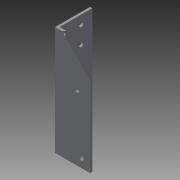
# Autodesk Inventor part: 2x2 angle vertical left
Saved by Autodesk Inventor 2015 (Build 190159000, 159)
## iProperties
Created: 2015-01-16
Part Number: 2x2 angle vertical left
Material: Generic
Document SubType Name: Modeling
Designer: 215152
Density: 1 g/cm^3
Appearance: Default
Author: 215152
Autodesk Inventor part; units mm, degrees
ref_plane "YZ Plane" through (0, 0, 0) normal (1, 0, 0) x (0, 1, 0)
ref_plane "XZ Plane" through (0, 0, 0) normal (0, 1, 0) x (-1, 0, 0)
ref_plane "XY Plane" through (0, 0, 0) normal (0, 0, 1) x (1, 0, 0)
sketch "Sketch1" plane through (0, 0, 0) normal (0, 1, 0) x (-1, 0, 0)
  line L0 (0, 0) -> (-3.175, 0)
  line L1 (-3.175, 0) -> (-3.175, -50.8)
  line L2 (-3.175, -50.8) -> (0, -50.8)
  line L3 (0, -50.8) -> (0, 0)
  line L4 (0, 0) -> (-50.8, 0)
  line L5 (-50.8, 0) -> (-50.8, -3.175)
  line L6 (-50.8, -3.175) -> (0, -3.175)
  line L7 (0, -3.175) -> (0, 0)
  dimension "d0" = 3.175
  dimension "d1" = 50.8
  dimension "d2" = 50.8
  dimension "d3" = 3.175
  constraints: 16 end point, 4 parallel, 2 horizontal, 2 perpendicular
  measures "d0" distance of L2.end L1.end
  measures "d1" distance of L1.end L0.end
  measures "d2" distance of L6.end L5.end
  measures "d3" distance of L5.end L4.end
extrude "Extrusion1" add sketch "Sketch1" along normal blind 158.75
sketch "Sketch2" plane through (0, 0, 0) normal (0, 0, 1) x (1, 0, 0)
  line L0 (0, 158.75) -> (50.8, 158.75) projected
  line L1 (0, 0) -> (0, 158.75) projected
  line L2 (0, 0) -> (50.8, 0) projected
  line L3 (50.8, 0) -> (50.8, 158.75) projected
  point P0 (31.75, 95.25)
  dimension "d6" = 31.75
  dimension "d7" = 63.5
  measures "d6" distance from line of L1 point (31.75, 95.25)
  measures "d7" distance from line of point (31.75, 95.25) L0
hole "Hole1" at (31.75, 95.25, 0) direction (0, 0, -1) diameter 6.35 end through all
sketch "Sketch3" plane through (0, 0, -50.8) normal (-1, 0, 0) x (0, 0, 1)
  line L0 (0, 0) -> (50.8, 0) projected
  line L1 (50.8, 0) -> (50.8, 158.75) projected
  line L2 (0, 158.75) -> (50.8, 158.75) projected
  line L3 (0, 0) -> (0, 158.75) projected
  point P0 (15.875, 146.05)
  point P1 (41.275, 146.05)
  point P2 (41.275, 120.65)
  point P3 (15.875, 120.65)
  dimension "d15" = 15.875
  dimension "d16" = 12.7
  dimension "d17" = 12.7
  dimension "d18" = 9.525
  dimension "d19" = 9.525
  dimension "d20" = 15.875
  dimension "d21" = 38.1
  dimension "d22" = 38.1
  measures "d15" distance from line of L3 point (15.875, 146.05)
  measures "d16" distance from line of L2 point (15.875, 146.05)
  measures "d17" distance from line of L2 point (41.275, 146.05)
  measures "d18" distance from line of L1 point (41.275, 146.05)
  measures "d19" distance from line of L1 point (41.275, 120.65)
  measures "d20" distance from line of L3 point (15.875, 120.65)
  measures "d21" distance from line of L2 point (15.875, 120.65)
  measures "d22" distance from line of L2 point (41.275, 120.65)
hole "Hole2" at (0, 146.05, -34.925) at (0, 146.05, -9.525) at (0, 120.65, -9.525) at (0, 120.65, -34.925) direction (1, 0, 0) diameter 6.35 end through all
sketch "Sketch4" plane through (0, 0, 0) normal (0, 0, 1) x (1, 0, 0)
  circle A0 centre (31.75, 95.25) radius 3.175 projected
  line L0 (0, 158.75) -> (50.8, 158.75) projected
  line L1 (0, 0) -> (0, 158.75) projected
  line L2 (0, 0) -> (50.8, 0) projected
  line L3 (50.8, 0) -> (50.8, 158.75) projected
  point P0 (38.1, 12.7)
  dimension "d30" = 12.7
  dimension "d31" = 12.7
  measures "d30" distance from line of L3 point (38.1, 12.7)
  measures "d31" distance from line of L2 point (38.1, 12.7)
hole "Hole3" at (38.1, 12.7, 0) direction (0, 0, -1) diameter 6.35 end through all
body "Solid1"
